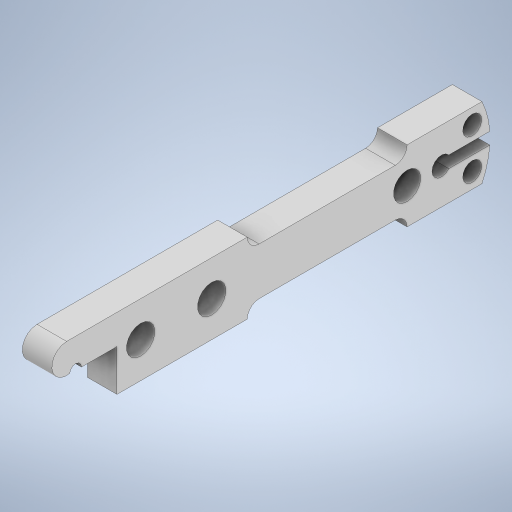
# Autodesk Inventor part: task5
Saved by Autodesk Inventor 2024.2 (Build 282272000, 272)
## iProperties
Created: 2024-11-03
Part Number: task5
Material: Типовые
Document SubType Name: Modeling
Designer: user
Density: 1 g/cm^3
Appearance: По умолчанию
Author: user
Autodesk Inventor part; units mm, degrees
ref_plane "YZ Plane" through (0, 0, 0) normal (1, 0, 0) x (0, 1, 0)
ref_plane "XZ Plane" through (0, 0, 0) normal (0, 1, 0) x (-1, 0, 0)
ref_plane "XY Plane" through (0, 0, 0) normal (0, 0, 1) x (1, 0, 0)
sketch "Эскиз1" plane through (0, 0, 0) normal (1, 0, 0) x (0, 1, 0)
  line L0 (2, -22) -> (-12, -22)
  line L1 (-12, -22) -> (-12, -66)
  line L2 (-12, -66) -> (-12, -66)
  line L3 (-8, -70) -> (-8, -116)
  line L4 (-12, -120) -> (-12, -120)
  line L5 (-12, -120) -> (-12, -142)
  line L6 (12, -142) -> (12, -120)
  line L7 (12, -120) -> (12, -120)
  line L8 (8, -116) -> (8, -70)
  line L9 (12, -66) -> (12, -66)
  line L10 (12, -66) -> (12, -8)
  arc A0 (2, -10) -> (2, -6) centre (2, -8) ccw
  line L11 (2, -10) -> (2, -22)
  line L12 (-12, -22) -> (-12, -30)
  circle A1 centre (0, -30) radius 4.8
  circle A2 centre (0, -54) radius 4.8
  circle A3 centre (0, -120) radius 4.6
  arc A4 (12, -66) -> (8, -70) centre (12, -70) ccw
  arc A5 (8, -116) -> (12, -120) centre (12, -116) ccw
  arc A6 (-12, -120) -> (-8, -116) centre (-12, -116) ccw
  arc A7 (-8, -70) -> (-12, -66) centre (-12, -70) ccw
  arc A8 (2, -134.098) -> (-2, -134.098) centre (0, -131.6) ccw
  circle A9 centre (-6.8, -142) radius 3.2
  circle A10 centre (6.8, -142) radius 3.2
  line L13 (-2, -142) -> (-2, -134.098)
  line L14 (2, -134.098) -> (2, -142)
  line L15 (12, -142) -> (12, -145.2982)
  line L16 (-12, -142) -> (-12, -145.2982)
  line L17 (2, -142) -> (2, -147.9285)
  line L18 (-2, -142) -> (-2, -147.9285)
  arc A11 (-12, -145.2982) -> (-2, -147.9285) centre (0, -120) ccw
  arc A12 (2, -147.9285) -> (12, -145.2982) centre (0, -120) ccw
  arc A13 (12, -5) -> (2.1015, -6.0026) centre (7, -5) ccw
  line L19 (12, -8) -> (12, -5)
  point P0 (0, 0)
  point P1 (8, -120)
  constraints: 40 end point, 19 point on circle, 14 centre point, 9 tangent, 7 point on line, 6 perpendicular, 6 vertical, 3 equal radius, 1 coincident
extrude "Выдавливание1" add sketch "Эскиз1" along normal blind 10
